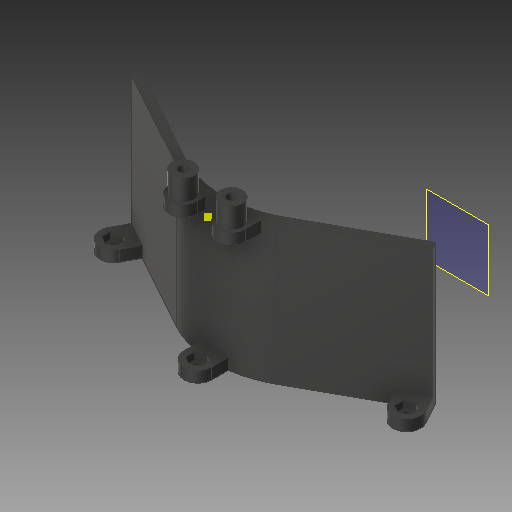
# Autodesk Inventor part: Capture Zone
Saved by Autodesk Inventor 2018 (Build 220112000, 112)
## iProperties
Created: 2018-06-13
Part Number: Capture Zone
Material: Acetal Resin, Black
Document SubType Name: Modeling
Designer: matth
Density: 1.425 g/cm^3
Appearance: Smooth - Black
Author: matth
Autodesk Inventor part; units mm, degrees
note: some values were not read from the file. Chosen so that the rebuilt part matches the saved one: direction of "Emboss1".
ref_plane "YZ Plane" through (0, 0, 0) normal (1, 0, 0) x (0, 1, 0)
ref_plane "XZ Plane" through (0, 0, 0) normal (0, 1, 0) x (-1, 0, 0)
ref_plane "XY Plane" through (0, 0, 0) normal (0, 0, 1) x (1, 0, 0)
sketch "Sketch1" plane through (0, 0, 0) normal (0, 1, 0) x (-1, 0, 0)
  line L0 (0, 0) -> (101.6431, 0) construction
  line L1 (0, 0) -> (-60.351, -33.192)
  line L2 (-60.351, -33.192) -> (60.351, -33.192)
  line L3 (60.351, -33.192) -> (0, 0)
  line L4 (-60.351, -33.192) -> (-61.7967, -30.5633)
  line L5 (-61.7967, -30.5633) -> (0, 3.4238)
  line L6 (60.351, -33.192) -> (61.7967, -30.5633)
  line L7 (61.7967, -30.5633) -> (0, 3.4238)
  dimension "d1" = 68.8763
  dimension "d2" = 120.702
  dimension "d3" = 3
  dimension "d4" = 3
  constraints: 16 end point, 2 perpendicular, 1 horizontal
  measures "d1" distance of L0.start L1.end
  measures "d2" distance of L1.end L2.end
  measures "d3" distance of L1.end L4.end
  measures "d4" distance of L2.end L6.end
extrude "Extrusion1" add sketch "Sketch1" along normal blind 50 contours L1 L4 L5 L7 L6 L3
fillet "Fillet1" radius 37 2 edges at (0, 25, 3.4238) (0, 25, 0)
sketch "Sketch5" plane through (0, 0, 0) normal (0, -1, 0) x (1, 0, 0)
  arc A0 (17.8305, -9.8065) -> (-17.8305, -9.8065) centre (0, -42.2267) ccw projected
  line L0 (0, -5.2267) -> (0, 3.7733)
  circle A1 centre (0, 3.7733) radius 1.75
  line L1 (0, 3.7733) -> (52.4, 3.7733)
  line L2 (52.4, 3.7733) -> (52.4, -18.5487)
  line L3 (52.4, 3.7733) -> (-52.4, 3.7733)
  line L4 (-52.4, 3.7733) -> (-52.4, -18.5487)
  circle A2 centre (-52.4, -18.5487) radius 1.75
  circle A3 centre (52.4, -18.5487) radius 1.75
  circle A4 centre (0, 3.7733) radius 5
  circle A5 centre (52.4, -18.5487) radius 5
  circle A6 centre (-52.4, -18.5487) radius 5
  line L5 (-5, 3.7733) -> (-5, -2.9446)
  line L6 (-5, -2.9446) -> (5, -2.9446)
  line L7 (5, -2.9446) -> (5, 3.7733)
  line L8 (52.4, -18.5487) -> (49.509, -23.8053)
  line L9 (17.8305, -6.3827) -> (61.7967, -30.5633) projected
  line L10 (49.509, -23.8053) -> (53.8901, -26.2148)
  line L11 (53.8901, -26.2148) -> (56.7811, -20.9582)
  line L12 (56.7811, -20.9582) -> (48.0189, -16.1392)
  line L13 (48.0189, -16.1392) -> (45.1279, -21.3957)
  line L14 (45.1279, -21.3957) -> (49.509, -23.8053)
  line L15 (-52.4, -18.5487) -> (-49.509, -23.8053)
  line L16 (-61.7967, -30.5633) -> (-17.8305, -6.3827) projected
  line L17 (-49.509, -23.8053) -> (-45.1279, -21.3957)
  line L18 (-45.1279, -21.3957) -> (-48.0189, -16.1392)
  line L19 (-48.0189, -16.1392) -> (-56.7811, -20.9582)
  line L20 (-56.7811, -20.9582) -> (-53.8901, -26.2148)
  line L21 (-53.8901, -26.2148) -> (-49.509, -23.8053)
  point P0 (0, 0)
  dimension "d30" = 9
  dimension "d31" = 3.5
  dimension "d32" = 52.4
  dimension "d33" = 22.322
  dimension "d34" = 104.8
  dimension "d35" = 3.5
  dimension "d36" = 3.5
  dimension "d37" = 10
  dimension "d38" = 10
  dimension "d39" = 10
  dimension "d40" = 5
  dimension "d41" = 5
  constraints: 40 end point, 11 perpendicular, 7 point on circle, 6 centre point, 6 coincident, 6 point on line, 3 vertical, 2 horizontal, 1 collinear, 1 tangent
  measures "d30" distance of L0.start L0.end
  measures "d31" diameter of A1
  measures "d32" distance of L1.start L1.end
  measures "d33" distance of L1.end L2.end
  measures "d34" distance of L1.end L3.end
  measures "d35" diameter of A2
  measures "d36" diameter of A3
  measures "d37" diameter of A4
  measures "d38" diameter of A5
  measures "d39" diameter of A6
  measures "d40" distance of L8.end L10.end
  measures "d41" distance of L15.end L17.end
extrude "Extrusion4" add sketch "Sketch5" against normal blind 4
sketch "Sketch6" plane through (0, 0, 0) normal (0, -1, 0) x (1, 0, 0)
  arc A0 (5, 3.7733) -> (-5, 3.7733) centre (0, 3.7733) ccw projected
  circle A1 centre (0, 3.7733) radius 1.75
  arc A2 (56.7811, -20.9582) -> (48.0189, -16.1392) centre (52.4, -18.5487) ccw projected
  circle A3 centre (52.4, -18.5487) radius 1.75
  arc A4 (-48.0189, -16.1392) -> (-56.7811, -20.9582) centre (-52.4, -18.5487) ccw projected
  circle A5 centre (-52.4, -18.5487) radius 1.75
  point P0 (0, 0)
  dimension "d44" = 3.5
  dimension "d45" = 3.5
  dimension "d46" = 3.5
  constraints: 3 centre point, 3 coincident
  measures "d44" diameter of A1
  measures "d45" diameter of A3
  measures "d46" diameter of A5
extrude "Extrusion5" cut sketch "Sketch6" against normal blind 4
sketch "Sketch7" plane through (0, 0, 0) normal (0, -1, 0) x (1, 0, 0)
  line L0 (-56.7811, -20.9582) -> (-53.8901, -26.2148) projected
  line L1 (-17.8305, -9.8065) -> (-60.351, -33.192) projected
  line L2 (-53.8901, -26.2148) -> (-52.4444, -28.8435)
  line L3 (-52.4444, -28.8435) -> (-60.351, -33.192)
  line L4 (-60.351, -33.192) -> (-61.7967, -30.5633)
  line L5 (-61.7967, -30.5633) -> (-53.8901, -26.2148)
  line L6 (53.8901, -26.2148) -> (61.7967, -30.5633) projected
  line L7 (53.8901, -26.2148) -> (61.7967, -30.5633)
  line L8 (61.7967, -30.5633) -> (60.351, -33.192)
  line L9 (60.351, -33.192) -> (52.4444, -28.8435)
  line L10 (52.4444, -28.8435) -> (53.8901, -26.2148)
  point P0 (0, 0)
  constraints: 16 end point, 5 equal length, 2 perpendicular, 1 point on line
extrude "Extrusion6" cut sketch "Sketch7" against normal blind 50
ref_plane "Work Plane2" through (56.4169, 50, -32.779) normal (0, 0, -1) x (-1, 0, 0)
sketch "Sketch10" plane through (56.4169, 50, -32.779) normal (0, 0, -1) x (-1, 0, 0)
  line L0 (20.4169, -11) -> (92.4169, -11) construction
  line L1 (92.4169, -11) -> (92.4169, -39) construction
  line L2 (92.4169, -39) -> (20.4169, -39) construction
  line L3 (20.4169, -39) -> (20.4169, -11) construction
  line L4 (108.8613, -50) -> (108.8613, 0) projected
  line L5 (3.9725, 0) -> (3.9725, -50) projected
  line L6 (105.9076, 0) -> (108.8613, 0) projected
  line L7 (74.2475, -50) -> (108.8613, -50) projected
  line L8 (44.3837, -36.5267) -> (41.0612, -36.5267)
  line L9 (41.0612, -36.5267) -> (41.0612, -14.9911)
  line L10 (41.0612, -14.9911) -> (34.5377, -29.6386)
  line L11 (34.5377, -29.6386) -> (32.5117, -29.6386)
  line L12 (32.5117, -29.6386) -> (26.049, -14.9911)
  line L13 (26.049, -14.9911) -> (26.049, -36.5267)
  line L14 (26.049, -36.5267) -> (22.9493, -36.5267)
  line L15 (22.9493, -36.5267) -> (22.9493, -11.5267)
  line L16 (22.9493, -11.5267) -> (27.4874, -11.5267)
  line L17 (27.4874, -11.5267) -> (33.7273, -25.4449)
  line L18 (33.7273, -25.4449) -> (39.7646, -11.5267)
  line L19 (39.7646, -11.5267) -> (44.3837, -11.5267)
  line L20 (44.3837, -11.5267) -> (44.3837, -36.5267)
  line L21 (71.1665, -36.5267) -> (66.8715, -36.5267)
  line L22 (66.8715, -36.5267) -> (63.4477, -32.9408)
  spline S0 degree 2 poles (63.4477, -32.9408) (61.7459, -35.1288) (58.1398, -37.0535) (55.8505, -37.0535) knots 0 0 0 1 2 2 2
  spline S1 degree 2 poles (55.8505, -37.0535) (52.4672, -37.0535) (48.0506, -32.9611) (48.0506, -29.6588) knots 0 0 0 1 2 2 2
  spline S2 degree 2 poles (48.0506, -29.6588) (48.0506, -28.2204) (48.861, -25.9716) (49.5296, -25.06) knots 0 0 0 1 2 2 2
  spline S3 degree 2 poles (49.5296, -25.06) (50.1779, -24.1888) (51.8999, -22.8517) (52.6698, -22.3655) knots 0 0 0 1 2 2 2
  spline S4 degree 2 poles (52.6698, -22.3655) (50.9882, -21.231) (49.3067, -18.6985) (49.3067, -16.7942) knots 0 0 0 1 2 2 2
  spline S5 degree 2 poles (49.3067, -16.7942) (49.3067, -15.5989) (50.2589, -13.5729) (51.0288, -12.8031) knots 0 0 0 1 2 2 2
  spline S6 degree 2 poles (51.0288, -12.8031) (51.8391, -12.013) (54.4121, -11) (55.9315, -11) knots 0 0 0 1 2 2 2
  spline S7 degree 2 poles (55.9315, -11) (58.7273, -11) (62.2524, -13.9376) (62.2524, -16.1864) knots 0 0 0 1 2 2 2
  spline S8 degree 2 poles (62.2524, -16.1864) (62.2524, -17.017) (61.827, -18.7796) (61.28, -19.5899) knots 0 0 0 1 2 2 2
  spline S9 degree 2 poles (61.28, -19.5899) (60.7127, -20.4206) (58.9299, -21.859) (57.4307, -22.406) knots 0 0 0 1 2 2 2
  line L23 (57.4307, -22.406) -> (63.3262, -28.4838)
  spline S10 degree 2 poles (63.3262, -28.4838) (63.549, -27.1062) (63.6503, -23.8647) (63.6503, -21.2512) knots 0 0 0 1 2 2 2
  line L24 (63.6503, -21.2512) -> (66.9323, -21.2512)
  line L25 (66.9323, -21.2512) -> (66.9323, -22.872)
  spline S11 degree 2 poles (66.9323, -22.872) (66.9323, -24.4724) (66.122, -28.5243) (65.1698, -30.3476) knots 0 0 0 1 2 2 2
  line L26 (65.1698, -30.3476) -> (71.1665, -36.5267)
  line L27 (61.9891, -31.4619) -> (54.2703, -23.5608)
  spline S12 degree 2 poles (54.2703, -23.5608) (53.8651, -23.8241) (53.0344, -24.5737) (52.528, -25.3031) knots 0 0 0 1 2 2 2
  spline S13 degree 2 poles (52.528, -25.3031) (52.1228, -25.8906) (51.515, -27.795) (51.515, -28.8485) knots 0 0 0 1 2 2 2
  spline S14 degree 2 poles (51.515, -28.8485) (51.515, -31.2391) (54.3513, -34.3185) (56.7621, -34.3185) knots 0 0 0 1 2 2 2
  spline S15 degree 2 poles (56.7621, -34.3185) (58.3626, -34.3185) (60.9356, -32.9611) (61.9891, -31.4619) knots 0 0 0 1 2 2 2
  spline S16 degree 2 poles (55.8505, -21.2107) (56.7824, -20.8865) (58.0182, -19.8128) (58.3626, -19.1848) knots 0 0 0 1 2 2 2
  spline S17 degree 2 poles (58.3626, -19.1848) (58.6665, -18.5972) (58.9704, -17.2804) (58.9704, -16.5105) knots 0 0 0 1 2 2 2
  spline S18 degree 2 poles (58.9704, -16.5105) (58.9704, -14.8898) (57.066, -13.107) (55.81, -13.107) knots 0 0 0 1 2 2 2
  spline S19 degree 2 poles (55.81, -13.107) (54.3108, -13.107) (52.5887, -15.1329) (52.5887, -16.6321) knots 0 0 0 1 2 2 2
  spline S20 degree 2 poles (52.5887, -16.6321) (52.5887, -17.3006) (52.8318, -18.2731) (53.237, -18.9011) knots 0 0 0 1 2 2 2
  spline S21 degree 2 poles (53.237, -18.9011) (53.6017, -19.4279) (54.8578, -20.6029) (55.8505, -21.2107) knots 0 0 0 1 2 2 2
  line L28 (69.9104, -36.5267) -> (78.3383, -11.5267)
  line L29 (78.3383, -11.5267) -> (82.4307, -11.5267)
  line L30 (82.4307, -11.5267) -> (90.8586, -36.5267)
  line L31 (90.8586, -36.5267) -> (87.3537, -36.5267)
  line L32 (87.3537, -36.5267) -> (85.0847, -29.5373)
  line L33 (85.0847, -29.5373) -> (75.5425, -29.5373)
  line L34 (75.5425, -29.5373) -> (73.2735, -36.5267)
  line L35 (73.2735, -36.5267) -> (69.9104, -36.5267)
  line L36 (84.173, -26.701) -> (80.3035, -14.9303)
  line L37 (80.3035, -14.9303) -> (76.4542, -26.701)
  line L38 (76.4542, -26.701) -> (84.173, -26.701)
  point P0 (56.4169, -50)
  dimension "d64" = 72
  dimension "d65" = 104.8888
  dimension "d66" = 16.4444
  dimension "d67" = 28
  dimension "d68" = 50
  dimension "d69" = 11
  constraints: 2 other
  measures "d64" distance of L1.end L2.end
  measures "d65" distance between parallel lines of L4 L5
  measures "d66" distance between parallel lines of L4 L1
  measures "d67" distance of L0.end L1.end
  measures "d68" distance between parallel lines of L6 L7
  measures "d69" distance between parallel lines of L6 L0
emboss "Emboss1" sketch "Sketch10" operation cut depth 0.5 direction (0, 0, 1)
sketch "Sketch16" plane through (0, 50, 0) normal (0, 1, 0) x (1, 0, 0)
  arc A0 (-17.8305, 9.8065) -> (17.8305, 9.8065) centre (0, 42.2267) ccw projected
  line L0 (0, 5.2267) -> (0, -1.0433)
  line L1 (0, -1.0433) -> (-8, -1.0433)
  line L2 (0, -1.0433) -> (9.27, -1.0433)
  circle A1 centre (9.27, -1.0433) radius 5
  circle A2 centre (-8, -1.0433) radius 5
  line L3 (14.27, -1.0433) -> (14.27, 5.6292)
  line L4 (14.27, 5.6292) -> (4.635, 4.4807)
  line L5 (4.635, 4.4807) -> (4.27, 3.2555)
  line L6 (4.27, 3.2555) -> (4.27, -1.0433)
  line L7 (-13, -1.0433) -> (-13, 6.0828)
  line L8 (-13, 6.0828) -> (-3, 3.5705)
  line L9 (-3, 3.5705) -> (-3, -1.0433)
  point P0 (0, 0)
  dimension "d85" = 6.27
  dimension "d86" = 8
  dimension "d87" = 9.27
  dimension "d88" = 10
  dimension "d89" = 10
  constraints: 20 end point, 5 point on circle, 3 vertical, 2 centre point, 2 coincident, 2 horizontal, 2 point on line
  measures "d85" distance of L0.start L0.end
  measures "d86" distance of L0.end L1.end
  measures "d87" distance of L0.end L2.end
  measures "d88" diameter of A1
  measures "d89" diameter of A2
extrude "Extrusion12" add sketch "Sketch16" against normal blind 4
sketch "Sketch17" plane through (0, 46, 0) normal (0, -1, 0) x (1, 0, 0)
  arc A0 (-3, 1.0433) -> (-13, 1.0433) centre (-8, 1.0433) ccw projected
  line L0 (-8, 1.0433) -> (-8, 4.2433)
  line L1 (-8, 1.0433) -> (-8, -2.1567)
  line L2 (-8, 1.0433) -> (-5.2287, 2.6433)
  line L3 (-8, 1.0433) -> (-4.8, 1.0433) construction
  line L4 (-8, 1.0433) -> (-5.2287, -0.5567)
  line L5 (-8, 1.0433) -> (-4.8, 1.0433) construction
  line L6 (-8, 1.0433) -> (-10.7713, 2.6433)
  line L7 (-8, 1.0433) -> (-10.7713, -0.5567)
  line L8 (-8, 4.2433) -> (-5.2287, 2.6433)
  line L9 (-5.2287, 2.6433) -> (-5.2287, -0.5567)
  line L10 (-5.2287, -0.5567) -> (-8, -2.1567)
  line L11 (-8, -2.1567) -> (-10.7713, -0.5567)
  line L12 (-10.7713, -0.5567) -> (-10.7713, 2.6433)
  line L13 (-10.7713, 2.6433) -> (-8, 4.2433)
  arc A1 (14.27, 1.0433) -> (4.27, 1.0433) centre (9.27, 1.0433) ccw projected
  line L14 (9.27, 1.0433) -> (9.27, 4.2433)
  line L15 (9.27, 1.0433) -> (12.0413, 2.6433)
  line L16 (9.27, 1.0433) -> (12.47, 1.0433) construction
  line L17 (9.27, 1.0433) -> (12.0413, -0.5567)
  line L18 (9.27, 1.0433) -> (12.47, 1.0433) construction
  line L19 (9.27, 1.0433) -> (9.27, -2.1567)
  line L20 (9.27, 1.0433) -> (6.4987, 2.6433)
  line L21 (9.27, 1.0433) -> (6.4987, -0.5567)
  line L22 (6.4987, 2.6433) -> (9.27, 4.2433)
  line L23 (9.27, 4.2433) -> (12.0413, 2.6433)
  line L24 (12.0413, 2.6433) -> (12.0413, -0.5567)
  line L25 (12.0413, -0.5567) -> (9.27, -2.1567)
  line L26 (9.27, -2.1567) -> (6.4987, -0.5567)
  line L27 (6.4987, -0.5567) -> (6.4987, 2.6433)
  point P0 (0, 0)
  dimension "d92" = 3.2
  dimension "d93" = 3.2
  dimension "d94" = 3.2
  dimension "d95" = 30
  dimension "d96" = 3.2
  dimension "d97" = 30
  dimension "d98" = 3.2
  dimension "d99" = 3.2
  dimension "d100" = 30
  dimension "d101" = 3.2
  dimension "d102" = 30
  dimension "d103" = 3.2
  constraints: 56 end point, 6 parallel, 4 equal length, 4 horizontal, 4 vertical, 1 point on line
  measures "d92" distance of L0.start L0.end
  measures "d93" distance of L0.start L1.end
  measures "d94" distance of L0.start L2.end
  measures "d95" angle of L3 L2
  measures "d96" distance of L0.start L4.end
  measures "d97" angle of L4 L5
  measures "d98" distance of L14.start L14.end
  measures "d99" distance of L14.start L15.end
  measures "d100" angle of L16 L15
  measures "d101" distance of L14.start L17.end
  measures "d102" angle of L17 L18
  measures "d103" distance of L14.start L19.end
extrude "Extrusion13" cut sketch "Sketch17" against normal blind 2.5
sketch "Sketch18" plane through (0, 50, 0) normal (0, 1, 0) x (1, 0, 0)
  arc A0 (4.27, -1.0433) -> (14.27, -1.0433) centre (9.27, -1.0433) ccw projected
  circle A1 centre (9.27, -1.0433) radius 4
  arc A2 (-13, -1.0433) -> (-3, -1.0433) centre (-8, -1.0433) ccw projected
  circle A3 centre (-8, -1.0433) radius 4
  point P0 (0, 0)
  dimension "d106" = 8
  dimension "d107" = 8
  constraints: 2 centre point, 2 coincident
  measures "d106" diameter of A1
  measures "d107" diameter of A3
extrude "Extrusion14" add sketch "Sketch18" along normal blind 7.5
sketch "Sketch19" plane through (9.27, 57.5, 1.0433) normal (0, 1, 0) x (1, 0, 0)
  circle A0 centre (0, 0) radius 4 projected
  circle A1 centre (0, 0) radius 1.75
  circle A2 centre (-17.27, 0) radius 4 projected
  circle A3 centre (-17.27, 0) radius 1.75
  point P0 (-9.27, 1.0433)
  dimension "d110" = 3.5
  dimension "d111" = 3.5
  constraints: 2 centre point, 2 coincident
  measures "d110" diameter of A1
  measures "d111" diameter of A3
extrude "Extrusion15" cut sketch "Sketch19" against normal blind 9 contours A1 | A3
sketch "Sketch21" plane through (0, 4, 0) normal (0, 1, 0) x (1, 0, 0)
  circle A0 centre (52.4, 18.5487) radius 1.75 projected
  line L0 (52.4, 18.5487) -> (52.4, 15.3487)
  line L1 (52.4, 18.5487) -> (52.4, 21.7487)
  line L2 (52.4, 18.5487) -> (49.6287, 20.1487)
  line L3 (52.4, 18.5487) -> (49.6287, 16.9487)
  line L4 (52.4, 18.5487) -> (55.6, 18.5487) construction
  line L5 (52.4, 18.5487) -> (55.1713, 16.9487)
  line L6 (52.4, 18.5487) -> (55.1713, 20.1487)
  line L7 (55.1713, 20.1487) -> (52.4, 21.7487)
  line L8 (52.4, 21.7487) -> (49.6287, 20.1487)
  line L9 (49.6287, 20.1487) -> (49.6287, 16.9487)
  line L10 (49.6287, 16.9487) -> (52.4, 15.3487)
  line L11 (52.4, 15.3487) -> (55.1713, 16.9487)
  line L12 (55.1713, 16.9487) -> (55.1713, 20.1487)
  point P0 (0, 0)
  dimension "d114" = 3.2
  dimension "d115" = 3.2
  dimension "d116" = 3.2
  dimension "d117" = 3.2
  dimension "d118" = 150
  constraints: 26 end point, 3 parallel, 3 vertical, 1 equal length, 1 horizontal
  measures "d114" distance of L0.start L0.end
  measures "d115" distance of L0.start L1.end
  measures "d116" distance of L0.start L2.end
  measures "d117" distance of L0.start L3.end
  measures "d118" angle of L3 L4
extrude "Extrusion16" cut sketch "Sketch21" against normal blind 2.5
sketch "Sketch22" plane through (0, 4, 0) normal (0, 1, 0) x (1, 0, 0)
  circle A0 centre (0, -3.7733) radius 1.75 projected
  line L0 (0, -3.7733) -> (0, -6.9733)
  line L1 (0, -6.9733) -> (-2.7713, -5.3733)
  line L2 (-2.7713, -5.3733) -> (-2.7713, -2.1733)
  line L3 (-2.7713, -2.1733) -> (0, -0.5733)
  line L4 (0, -0.5733) -> (2.7713, -2.1733)
  line L5 (2.7713, -2.1733) -> (2.7713, -5.3733)
  line L6 (2.7713, -5.3733) -> (0, -6.9733)
  circle A1 centre (-52.4, 18.5487) radius 1.75 projected
  line L7 (-52.4, 18.5487) -> (-52.4, 15.3487)
  line L8 (-52.4, 15.3487) -> (-55.1713, 16.9487)
  line L9 (-55.1713, 16.9487) -> (-55.1713, 20.1487)
  line L10 (-55.1713, 20.1487) -> (-52.4, 21.7487)
  line L11 (-52.4, 21.7487) -> (-49.6287, 20.1487)
  line L12 (-49.6287, 20.1487) -> (-49.6287, 16.9487)
  line L13 (-49.6287, 16.9487) -> (-52.4, 15.3487)
  point P0 (0, 0)
  dimension "d121" = 3.2
  dimension "d122" = 3.2
  dimension "d123" = 60
  dimension "d124" = 3.2
  dimension "d125" = 3.2
  dimension "d126" = 3.2
  dimension "d127" = 60
  dimension "d128" = 3.2
  constraints: 28 end point, 8 parallel, 2 vertical
  measures "d121" distance of L0.start L0.end
  measures "d122" distance of L0.end L1.end
  measures "d123" angle of L0 L1
  measures "d124" distance of L1.end L2.end
  measures "d125" distance of L7.start L7.end
  measures "d126" distance of L7.end L8.end
  measures "d127" angle of L7 L8
  measures "d128" distance of L8.end L9.end
extrude "Extrusion17" cut sketch "Sketch22" against normal blind 2.5
sketch "Sketch23" plane through (0, 46, 0) normal (0, -1, 0) x (1, 0, 0)
  point P0 (0, 0)
equation "\"d66\" = -0.5 * d64 + 0.5 * d65"
equation "\"d69\" = -0.5 * d67 + 0.5 * d68"
body "Solid1"
